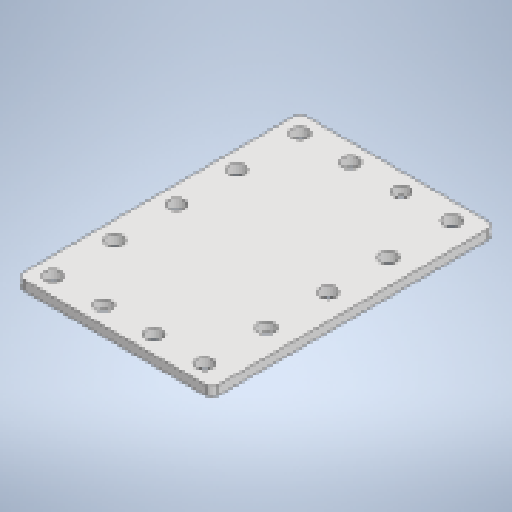
# Autodesk Inventor part: PRS 1200-07 charging flange rect
Saved by Autodesk Inventor 2025.4 (Build 294407000, 407)
## iProperties
Created: 2025-02-13
Part Number: PRS 1200-07 charging flange rect
Material: Steel
Document SubType Name: Sheet Metal
Designer: admin
Mass: 2466.79 g
Surface Area: 934.137 cm^2
Volume: 314.241 cm^3
Density: 7.85 g/cm^3
Flat Pattern Width: 30.2 cm
Flat Pattern Length: 20.8 cm
Flat Pattern Area: 628.16 cm^2
Sheet Metal Rule: AISI304 4mm Die 32
Sheet Metal Width: 302,000 mm
Sheet Metal Length: 208,000 mm
Sheet Metal Area: 62816,000 mm^2
Appearance: Default
Author: pokla
Autodesk Inventor part; units mm, degrees
ref_plane "YZ Plane" through (0, 0, 0) normal (1, 0, 0) x (0, 1, 0)
ref_plane "XZ Plane" through (0, 0, 0) normal (0, 1, 0) x (-1, 0, 0)
ref_plane "XY Plane" through (0, 0, 0) normal (0, 0, 1) x (1, 0, 0)
sketch "Sketch2" plane through (0, 0, 0) normal (0, 0, 1) x (1, 0, 0)
  line L0 (-54, -101) -> (54, -101)
  line L1 (54, -101) -> (54, 101)
  line L2 (54, 101) -> (-54, 101)
  line L3 (-54, 101) -> (-54, -101)
  line L4 (-54, -101) -> (54, 101) construction
  line L5 (54, -101) -> (-54, 101) construction
  line L6 (-104, -151) -> (104, -151)
  line L7 (104, -151) -> (104, 151)
  line L8 (104, 151) -> (-104, 151)
  line L9 (-104, 151) -> (-104, -151)
  point P0 (0, 0)
  dimension "d29" = 108
  dimension "d30" = 202
  dimension "d31" = 50
  measures "d29" distance of L2.end L1.end
  measures "d30" distance of L1.end L0.end
  measures "d31" distance between parallel lines of L3 L9
extrude "Plate2" add sketch "Sketch2" along normal blind 10 contours L3 L2 L1 L0 | L9 L8 L7 L6
sketch "Sketch5" plane through (0, 0, 10) normal (0, 0, 1) x (1, 0, 0)
  line L0 (104, -151) -> (-104, -151) construction
  line L1 (104, 151) -> (104, -151) construction
  line L2 (-104, 151) -> (104, 151) construction
  line L3 (-104, -151) -> (-104, 151) construction
  line L4 (-85, 132) -> (85, 132) construction
  line L5 (85, 132) -> (85, -132) construction
  line L6 (85, -132) -> (-85, -132) construction
  line L7 (-85, -132) -> (-85, 132) construction
  circle A0 centre (-85, -132) radius 8.5
  circle A1 centre (-85, 132) radius 8.5
  circle A2 centre (-85, 0) radius 8.5
  circle A3 centre (-85, -66) radius 8.5
  circle A4 centre (-85, 64.5) radius 8.5
  line L8 (-50, -0.75) -> (50, -0.75) construction
  circle A5 centre (-31, -132) radius 8.5
  circle A6 centre (-31, -66) radius 8.5
  circle A7 centre (-31, 0) radius 8.5
  circle A8 centre (-31, 64.5) radius 8.5
  circle A9 centre (-31, 132) radius 8.5
  circle A10 centre (23, -132) radius 8.5
  circle A11 centre (23, -66) radius 8.5
  circle A12 centre (23, 0) radius 8.5
  circle A13 centre (23, 64.5) radius 8.5
  circle A14 centre (23, 132) radius 8.5
  circle A15 centre (77, -132) radius 8.5
  circle A16 centre (77, -66) radius 8.5
  circle A17 centre (77, 0) radius 8.5
  circle A18 centre (77, 64.5) radius 8.5
  circle A19 centre (77, 132) radius 8.5
  point P0 (0, 0)
  point P1 (0, -132)
  dimension "d33" = 17
  dimension "d34" = 19
  dimension "d35" = 66
  dimension "d36" = 66
  dimension "d39" = 54
  constraints: 20 centre point, 10 end point, 8 coincident, 4 equal radius, 2 midpoint, 2 point on line, 1 horizontal, 40 other
  measures "d33" diameter of A0
  measures "d34" distance between parallel lines of L0 L6
  measures "d35" distance of A3.centre L6.end
  measures "d36" distance of A3.centre A2.centre
  measures "d39" distance of L6.end point (-31, -132)
extrude "Cut3" cut sketch "Sketch5" against normal blind 10 contours A0 | A1 | A2 | A3 | A4 | A5 | A9 | A10 | A14 | A15 | A16 | A17 | A18 | A19
fillet "Corner Round1" radius 6 4 edges at (-104, -151, 5) (-104, 151, 5) (104, 151, 5) (104, -151, 5)
equation "\"d35\" = d36"
equation "\"d44\" = Thickness"
equation "\"d14\" = Thickness"
equation "\"BendReliefDepth\" = 0.5 * Thickness"
equation "\"TransitionRadius\" = BendRadius"
equation "\"JacobiRadiusSize\" = BendRadius"
equation "\"Thickness\" = 10"
equation "\"BendRadius\" = 6"
body "Solid3"
